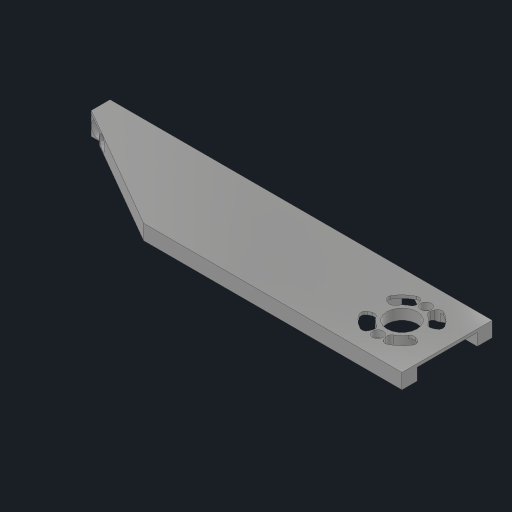
# Autodesk Inventor part: right_hold
Saved by Autodesk Inventor 2023 (Build 270158000, 158)
## iProperties
Created: 2024-05-18
Part Number: right_hold
Material: Nylon 6/6
Document SubType Name: Modeling
Designer: szymo
Density: 1.13 g/cm^3
Appearance: Smooth - Medium Gray
Mass: 11.7755 g
Surface Area: 98.1718 cm^2
Volume: 10.4208 cm^3
Author: szymo
Autodesk Inventor part; units mm, degrees
ref_plane "YZ Plane" through (0, 0, 0) normal (1, 0, 0) x (0, 1, 0)
ref_plane "XZ Plane" through (0, 0, 0) normal (0, 1, 0) x (-1, 0, 0)
ref_plane "XY Plane" through (0, 0, 0) normal (0, 0, 1) x (1, 0, 0)
ref_plane "Work Plane1" through (0, 0, 0) normal (0, 0, 1) x (1, 0, 0)
sketch "Sketch1" plane through (0, 0, 0) normal (0, 0, 1) x (1, 0, 0)
  line L0 (-71, -74) -> (-71, -89) projected
  line L1 (-71, -89) -> (41, -89) projected
  line L2 (41, -89) -> (41, -30.5) projected
  line L3 (41, -30.5) -> (91, -30.5) projected
  line L4 (91, -30.5) -> (91, 30.5) projected
  line L5 (91, 30.5) -> (41, 30.5) projected
  line L6 (41, 30.5) -> (41, 89) projected
  line L7 (41, 89) -> (-71, 89) projected
  line L8 (-71, 89) -> (-71, 74) projected
  line L9 (-71, 74) -> (-87, 74) projected
  line L10 (-87, 74) -> (-87, 89) projected
  line L11 (-87, 89) -> (-91, 89) projected
  line L12 (-91, 89) -> (-91, -89) projected
  line L13 (-91, -89) -> (-87, -89) projected
  line L14 (-87, -89) -> (-87, -74) projected
  line L15 (-87, -74) -> (-71, -74) projected
  line L16 (12, 37) -> (40, 37) projected
  line L17 (41, 37) -> (-86, 37)
  line L18 (-86, 37) -> (-86, 36)
  line L19 (-86, 36) -> (41, 36)
  line L20 (41, 36) -> (41, 37)
  circle A0 centre (-83, 21.5) radius 1.2295 projected
  circle A1 centre (-83, -64.5) radius 1.2295 projected
  circle A2 centre (-83, -21.5) radius 1.2295 projected
  circle A3 centre (-83, 64.5) radius 1.2295 projected
  line L21 (-85, -72) -> (-76, -72) projected
  line L22 (-76, -72) -> (-76, -57) projected
  line L23 (-76, -57) -> (-85, -57) projected
  arc A4 (-87, -55) -> (-85, -57) centre (-85, -55) ccw projected
  line L24 (-87, -55) -> (-87, -31) projected
  arc A5 (-85, -29) -> (-87, -31) centre (-85, -31) ccw projected
  line L25 (-85, -29) -> (-76, -29) projected
  line L26 (-76, -29) -> (-76, -14) projected
  line L27 (-76, -14) -> (-85, -14) projected
  arc A6 (-87, -12) -> (-85, -14) centre (-85, -12) ccw projected
  line L28 (-87, -12) -> (-87, 12) projected
  arc A7 (-85, 14) -> (-87, 12) centre (-85, 12) ccw projected
  line L29 (-85, 14) -> (-76, 14) projected
  line L30 (-76, 14) -> (-76, 29) projected
  line L31 (-76, 29) -> (-85, 29) projected
  arc A8 (-87, 31) -> (-85, 29) centre (-85, 31) ccw projected
  line L32 (-87, 31) -> (-87, 55) projected
  arc A9 (-85, 57) -> (-87, 55) centre (-85, 55) ccw projected
  line L33 (-85, 57) -> (-76, 57) projected
  line L34 (-76, 57) -> (-76, 72) projected
  line L35 (-76, 72) -> (-85, 72) projected
  arc A10 (-87, 74) -> (-85, 72) centre (-85, 74) ccw projected
  line L36 (-87, 74) -> (-87, 89) projected
  line L37 (-91, 89) -> (-87, 89) projected
  line L38 (-91, -89) -> (-91, 89) projected
  line L39 (-91, -89) -> (-87, -89) projected
  line L40 (-87, -89) -> (-87, -74) projected
  arc A11 (-85, -72) -> (-87, -74) centre (-85, -74) ccw projected
  point P0 (0, 0)
  dimension "d1" = 0
  dimension "d2" = 1
  dimension "d11" = 1
  constraints: 8 end point, 2 parallel, 1 horizontal, 1 perpendicular, 1 point on line
  measures "d1" distance between parallel lines of L16 L17
  measures "d2" distance between parallel lines of L16 L19
  measures "d11" distance between parallel lines of L18 L32
ref_plane "Work Plane2" through (11, 8.5, 30) normal (0, 0, 1) x (1, 0, 0)
extrude "Extrusion1" add sketch "Sketch1" along normal up to surface (30 mm away) contours L19 L18 L17 L16 L6
ref_plane "Work Plane3" through (-90.5, 89, 1) normal (0, 1, 0) x (0, 0, 1)
sketch "Sketch3" plane through (-90.5, 89, 1) normal (0, 1, 0) x (0, 0, 1)
  line L0 (3.5, 3.5) -> (-1, 3.5) projected
  line L1 (-1, 3.5) -> (-1, -0.5) projected
  line L2 (-1, -0.5) -> (-4.5, -0.5) projected
  line L3 (-4.5, -0.5) -> (-4.5, -14.5) projected
  line L4 (-4.5, -14.5) -> (4.5, -0.5) projected
  line L5 (4.5, -0.5) -> (3.5, -0.5) projected
  line L6 (3.5, -0.5) -> (3.5, 3.5) projected
  line L7 (29, 4.5) -> (29, 131.5) projected
  line L8 (-1, 131.5) -> (29, 131.5) projected
  line L9 (-1, 131.5) -> (-1, 4.5) projected
  line L10 (-1, 4.5) -> (29, 4.5) projected
  line L11 (3.5, -0.5) -> (30.1547, 45.6673)
  line L12 (30.1547, 45.6673) -> (29, 45.6673)
  line L13 (29, 45.6673) -> (3.5, 1.5)
  point P0 (-1, 90.5)
  point P1 (5.2321, 4.5)
  dimension "d13" = 1
  constraints: 6 end point, 1 midpoint, 1 parallel, 1 perpendicular, 1 point on line
  measures "d13" distance between parallel lines of L13 L11
extrude "Extrusion3" cut sketch "Sketch3" against normal up to next contours L13 L7 L11 L10 | L11 L7 L10
sketch "Sketch7" plane through (41, 36, 0) normal (0, -1, 0) x (1, 0, 0)
  line L0 (-23.0542, 11.42) -> (-22.0416, 11.8701) projected
  arc A0 (-20.7815, 11.4767) -> (-22.0416, 11.8701) centre (-21.6354, 10.9563) ccw projected
  arc A1 (-20.7815, 11.4767) -> (-18.0539, 8.9574) centre (-15, 15) ccw projected
  arc A2 (-17.5618, 7.7324) -> (-18.0539, 8.9574) centre (-18.5049, 8.0649) ccw projected
  line L1 (-17.5618, 7.7324) -> (-17.9302, 6.6874) projected
  arc A3 (-19.3099, 6.1202) -> (-17.9302, 6.6874) centre (-18.8733, 7.0198) ccw projected
  arc A4 (-23.5102, 9.9996) -> (-19.3099, 6.1202) centre (-15, 15) ccw projected
  arc A5 (-23.0542, 11.42) -> (-23.5102, 9.9996) centre (-22.648, 10.5062) ccw projected
  line L2 (-7.9584, 11.8701) -> (-6.9458, 11.42) projected
  arc A6 (-6.4898, 9.9996) -> (-6.9458, 11.42) centre (-7.352, 10.5062) ccw projected
  arc A7 (-10.6901, 6.1202) -> (-6.4898, 9.9996) centre (-15, 15) ccw projected
  arc A8 (-12.0698, 6.6874) -> (-10.6901, 6.1202) centre (-11.1267, 7.0198) ccw projected
  line L3 (-12.0698, 6.6874) -> (-12.4382, 7.7324) projected
  arc A9 (-11.9461, 8.9574) -> (-12.4382, 7.7324) centre (-11.4951, 8.0649) ccw projected
  arc A10 (-11.9461, 8.9574) -> (-9.2185, 11.4767) centre (-15, 15) ccw projected
  arc A11 (-7.9584, 11.8701) -> (-9.2185, 11.4767) centre (-8.3646, 10.9563) ccw projected
  line L4 (-22.0416, 18.1299) -> (-23.0542, 18.58) projected
  arc A12 (-23.5102, 20.0004) -> (-23.0542, 18.58) centre (-22.648, 19.4938) ccw projected
  arc A13 (-19.3099, 23.8798) -> (-23.5102, 20.0004) centre (-15, 15) ccw projected
  arc A14 (-17.9302, 23.3126) -> (-19.3099, 23.8798) centre (-18.8733, 22.9802) ccw projected
  line L5 (-17.9302, 23.3126) -> (-17.5618, 22.2676) projected
  arc A15 (-18.0539, 21.0426) -> (-17.5618, 22.2676) centre (-18.5049, 21.9351) ccw projected
  arc A16 (-18.0539, 21.0426) -> (-20.7815, 18.5233) centre (-15, 15) ccw projected
  arc A17 (-22.0416, 18.1299) -> (-20.7815, 18.5233) centre (-21.6354, 19.0437) ccw projected
  line L6 (-6.9458, 18.58) -> (-7.9584, 18.1299) projected
  arc A18 (-9.2185, 18.5233) -> (-7.9584, 18.1299) centre (-8.3646, 19.0437) ccw projected
  arc A19 (-9.2185, 18.5233) -> (-11.9461, 21.0426) centre (-15, 15) ccw projected
  arc A20 (-12.4382, 22.2676) -> (-11.9461, 21.0426) centre (-11.4951, 21.9351) ccw projected
  line L7 (-12.4382, 22.2676) -> (-12.0698, 23.3126) projected
  arc A21 (-10.6901, 23.8798) -> (-12.0698, 23.3126) centre (-11.1267, 22.9802) ccw projected
  arc A22 (-6.4898, 20.0004) -> (-10.6901, 23.8798) centre (-15, 15) ccw projected
  arc A23 (-6.9458, 18.58) -> (-6.4898, 20.0004) centre (-7.352, 19.4938) ccw projected
  circle A24 centre (-15, 23) radius 1.2295 projected
  circle A25 centre (-15, 7) radius 1.2295 projected
  circle A26 centre (-15, 15) radius 5 projected
  circle A27 centre (-15, 15) radius 14 projected
  circle A28 centre (-15, 15) radius 15 projected
  arc A29 (-23.9413, 20.2537) -> (-23.2572, 18.1231) centre (-22.648, 19.4938) ccw
  line L8 (-23.2572, 18.1231) -> (-22.2447, 17.673)
  arc A30 (-22.2447, 17.673) -> (-20.3545, 18.2631) centre (-21.6354, 19.0437) ccw
  arc A31 (-17.8283, 20.5964) -> (-20.3545, 18.2631) centre (-15, 15) ccw
  arc A32 (-17.8283, 20.5964) -> (-17.0902, 22.4338) centre (-18.5049, 21.9351) ccw
  line L9 (-17.0902, 22.4338) -> (-17.4586, 23.4789)
  arc A33 (-17.4586, 23.4789) -> (-19.5283, 24.3296) centre (-18.8733, 22.9802) ccw
  arc A34 (-19.5283, 24.3296) -> (-23.9413, 20.2537) centre (-15, 15) ccw
  arc A35 (-10.4717, 24.3296) -> (-12.5414, 23.4789) centre (-11.1267, 22.9802) ccw
  line L10 (-12.5414, 23.4789) -> (-12.9098, 22.4338)
  arc A36 (-12.9098, 22.4338) -> (-12.1717, 20.5964) centre (-11.4951, 21.9351) ccw
  arc A37 (-9.6455, 18.2631) -> (-12.1717, 20.5964) centre (-15, 15) ccw
  arc A38 (-9.6455, 18.2631) -> (-7.7553, 17.673) centre (-8.3646, 19.0437) ccw
  line L11 (-7.7553, 17.673) -> (-6.7428, 18.1231)
  arc A39 (-6.7428, 18.1231) -> (-6.0587, 20.2537) centre (-7.352, 19.4938) ccw
  arc A40 (-6.0587, 20.2537) -> (-10.4717, 24.3296) centre (-15, 15) ccw
  arc A41 (-20.3545, 11.7369) -> (-17.8283, 9.4036) centre (-15, 15) ccw
  arc A42 (-20.3545, 11.7369) -> (-22.2447, 12.327) centre (-21.6354, 10.9563) ccw
  line L12 (-22.2447, 12.327) -> (-23.2572, 11.8769)
  arc A43 (-23.2572, 11.8769) -> (-23.9413, 9.7463) centre (-22.648, 10.5062) ccw
  arc A44 (-23.9413, 9.7463) -> (-19.5283, 5.6704) centre (-15, 15) ccw
  arc A45 (-19.5283, 5.6704) -> (-17.4586, 6.5211) centre (-18.8733, 7.0198) ccw
  line L13 (-17.4586, 6.5211) -> (-17.0902, 7.5662)
  arc A46 (-17.0902, 7.5662) -> (-17.8283, 9.4036) centre (-18.5049, 8.0649) ccw
  arc A47 (-12.1717, 9.4036) -> (-9.6455, 11.7369) centre (-15, 15) ccw
  arc A48 (-12.1717, 9.4036) -> (-12.9098, 7.5662) centre (-11.4951, 8.0649) ccw
  line L14 (-12.9098, 7.5662) -> (-12.5414, 6.5211)
  arc A49 (-12.5414, 6.5211) -> (-10.4717, 5.6704) centre (-11.1267, 7.0198) ccw
  arc A50 (-10.4717, 5.6704) -> (-6.0587, 9.7463) centre (-15, 15) ccw
  arc A51 (-6.0587, 9.7463) -> (-6.7428, 11.8769) centre (-7.352, 10.5062) ccw
  line L15 (-6.7428, 11.8769) -> (-7.7553, 12.327)
  arc A52 (-7.7553, 12.327) -> (-9.6455, 11.7369) centre (-8.3646, 10.9563) ccw
  circle A53 centre (-15, 23) radius 1.4
  circle A54 centre (-15, 7) radius 1.4
  point P0 (-41, 0)
  dimension "d21" = 0.5
  dimension "d22" = 0.5
  dimension "d23" = 0.5
  dimension "d24" = 0.5
  dimension "d25" = 2.8
  dimension "d26" = 2.8
  constraints: 48 point on circle, 26 centre point, 16 end point, 2 coincident, 28 other
  measures "d21" radial gap between concentric circles of A13 A34
  measures "d22" radial gap between concentric circles of A22 A40
  measures "d23" radial gap between concentric circles of A1 A41
  measures "d24" radial gap between concentric circles of A10 A47
  measures "d25" diameter of A53
  measures "d26" diameter of A54
extrude "motur" cut sketch "Sketch7" against normal up to next contours L0 A0 A1 A2 L1 A3 A4 A5 | L2 A6 A7 A8 L3 A9 A10 A11 | L4 A12 A13 A14 L5 A15 A16 A17 | L6 A18 A19 A20 L7 A21 A22 A23 | A24 | A25 | A26 | A34 A33 L9 A32 A31 A30 L8 A29 | A40 A39 L11 A38 A37 A36 L10 A35 | A41 A46 L13 A45 A44 A43 L12 A42 | A47 A52 L15 A51 A50 A49 L14 A48 | A53 | A54
sketch "Sketch9" plane through (-86, 36, 0) normal (0, -1, 0) x (1, 0, 0)
  circle A0 centre (112, 23) radius 1.4 projected
  arc A1 (103.0587, 9.7463) -> (107.4717, 5.6704) centre (112, 15) ccw projected
  arc A2 (103.7428, 11.8769) -> (103.0587, 9.7463) centre (104.352, 10.5062) ccw projected
  line L0 (103.7428, 11.8769) -> (104.7553, 12.327) projected
  arc A3 (106.6455, 11.7369) -> (104.7553, 12.327) centre (105.3646, 10.9563) ccw projected
  arc A4 (106.6455, 11.7369) -> (109.1717, 9.4036) centre (112, 15) ccw projected
  arc A5 (109.9098, 7.5662) -> (109.1717, 9.4036) centre (108.4951, 8.0649) ccw projected
  line L1 (109.9098, 7.5662) -> (109.5414, 6.5211) projected
  arc A6 (107.4717, 5.6704) -> (109.5414, 6.5211) centre (108.1267, 7.0198) ccw projected
  arc A7 (120.2572, 18.1231) -> (120.9413, 20.2537) centre (119.648, 19.4938) ccw projected
  line L2 (120.2572, 18.1231) -> (119.2447, 17.673) projected
  arc A8 (117.3545, 18.2631) -> (119.2447, 17.673) centre (118.6354, 19.0437) ccw projected
  arc A9 (117.3545, 18.2631) -> (114.8283, 20.5964) centre (112, 15) ccw projected
  arc A10 (114.0902, 22.4338) -> (114.8283, 20.5964) centre (115.5049, 21.9351) ccw projected
  line L3 (114.0902, 22.4338) -> (114.4586, 23.4789) projected
  arc A11 (116.5283, 24.3296) -> (114.4586, 23.4789) centre (115.8733, 22.9802) ccw projected
  arc A12 (120.9413, 20.2537) -> (116.5283, 24.3296) centre (112, 15) ccw projected
  arc A13 (109.5414, 23.4789) -> (107.4717, 24.3296) centre (108.1267, 22.9802) ccw projected
  line L4 (109.5414, 23.4789) -> (109.9098, 22.4338) projected
  arc A14 (109.1717, 20.5964) -> (109.9098, 22.4338) centre (108.4951, 21.9351) ccw projected
  arc A15 (109.1717, 20.5964) -> (106.6455, 18.2631) centre (112, 15) ccw projected
  arc A16 (104.7553, 17.673) -> (106.6455, 18.2631) centre (105.3646, 19.0437) ccw projected
  line L5 (104.7553, 17.673) -> (103.7428, 18.1231) projected
  arc A17 (103.0587, 20.2537) -> (103.7428, 18.1231) centre (104.352, 19.4938) ccw projected
  arc A18 (107.4717, 24.3296) -> (103.0587, 20.2537) centre (112, 15) ccw projected
  circle A19 centre (112, 7) radius 1.4 projected
  arc A20 (116.5283, 5.6704) -> (120.9413, 9.7463) centre (112, 15) ccw projected
  arc A21 (114.4586, 6.5211) -> (116.5283, 5.6704) centre (115.8733, 7.0198) ccw projected
  line L6 (114.4586, 6.5211) -> (114.0902, 7.5662) projected
  arc A22 (114.8283, 9.4036) -> (114.0902, 7.5662) centre (115.5049, 8.0649) ccw projected
  arc A23 (114.8283, 9.4036) -> (117.3545, 11.7369) centre (112, 15) ccw projected
  arc A24 (119.2447, 12.327) -> (117.3545, 11.7369) centre (118.6354, 10.9563) ccw projected
  line L7 (119.2447, 12.327) -> (120.2572, 11.8769) projected
  arc A25 (120.9413, 9.7463) -> (120.2572, 11.8769) centre (119.648, 10.5062) ccw projected
  circle A26 centre (112, 15) radius 5 projected
  line L8 (41.1673, 30) -> (0, 6.2321) projected
  line L9 (0, 0) -> (0, 6.2321) projected
  line L10 (0, 0) -> (127, 0) projected
  line L11 (127, 0) -> (127, 30) projected
  line L12 (127, 30) -> (41.1673, 30) projected
  line L13 (0, 6.2321) -> (6.5, 6.2321)
  line L14 (6.5, 6.2321) -> (6.5, 0)
  line L15 (6.5, 0) -> (0, 0)
  line L16 (0, 0) -> (0, 6.2321)
  point P0 (86, 0)
  dimension "d31" = 6.5
  constraints: 8 end point, 2 parallel, 1 horizontal, 1 perpendicular, 1 point on line
  measures "d31" distance of L14.end L15.end
extrude "forScrew" add sketch "Sketch9" along normal blind 6.5 contours L13 L14 L10 L9
sketch "Sketch10" plane through (41, 36, 0) normal (0, -1, 0) x (1, 0, 0)
  line L0 (-120.5, 6.2321) -> (-120.5, 0) projected
  line L1 (-120.5, 0) -> (0, 0) projected
  line L2 (0, 0) -> (0, 30) projected
  line L3 (0, 30) -> (-85.8327, 30) projected
  line L4 (-85.8327, 30) -> (-127, 6.2321) projected
  line L5 (-127, 6.2321) -> (-120.5, 6.2321) projected
  circle A0 centre (-15, 23) radius 1.4 projected
  arc A1 (-23.9413, 9.7463) -> (-19.5283, 5.6704) centre (-15, 15) ccw projected
  arc A2 (-23.2572, 11.8769) -> (-23.9413, 9.7463) centre (-22.648, 10.5062) ccw projected
  line L6 (-23.2572, 11.8769) -> (-22.2447, 12.327) projected
  arc A3 (-20.3545, 11.7369) -> (-22.2447, 12.327) centre (-21.6354, 10.9563) ccw projected
  arc A4 (-20.3545, 11.7369) -> (-17.8283, 9.4036) centre (-15, 15) ccw projected
  arc A5 (-17.0902, 7.5662) -> (-17.8283, 9.4036) centre (-18.5049, 8.0649) ccw projected
  line L7 (-17.0902, 7.5662) -> (-17.4586, 6.5211) projected
  arc A6 (-19.5283, 5.6704) -> (-17.4586, 6.5211) centre (-18.8733, 7.0198) ccw projected
  arc A7 (-6.7428, 18.1231) -> (-6.0587, 20.2537) centre (-7.352, 19.4938) ccw projected
  line L8 (-6.7428, 18.1231) -> (-7.7553, 17.673) projected
  arc A8 (-9.6455, 18.2631) -> (-7.7553, 17.673) centre (-8.3646, 19.0437) ccw projected
  arc A9 (-9.6455, 18.2631) -> (-12.1717, 20.5964) centre (-15, 15) ccw projected
  arc A10 (-12.9098, 22.4338) -> (-12.1717, 20.5964) centre (-11.4951, 21.9351) ccw projected
  line L9 (-12.9098, 22.4338) -> (-12.5414, 23.4789) projected
  arc A11 (-10.4717, 24.3296) -> (-12.5414, 23.4789) centre (-11.1267, 22.9802) ccw projected
  arc A12 (-6.0587, 20.2537) -> (-10.4717, 24.3296) centre (-15, 15) ccw projected
  arc A13 (-17.4586, 23.4789) -> (-19.5283, 24.3296) centre (-18.8733, 22.9802) ccw projected
  line L10 (-17.4586, 23.4789) -> (-17.0902, 22.4338) projected
  arc A14 (-17.8283, 20.5964) -> (-17.0902, 22.4338) centre (-18.5049, 21.9351) ccw projected
  arc A15 (-17.8283, 20.5964) -> (-20.3545, 18.2631) centre (-15, 15) ccw projected
  arc A16 (-22.2447, 17.673) -> (-20.3545, 18.2631) centre (-21.6354, 19.0437) ccw projected
  line L11 (-22.2447, 17.673) -> (-23.2572, 18.1231) projected
  arc A17 (-23.9413, 20.2537) -> (-23.2572, 18.1231) centre (-22.648, 19.4938) ccw projected
  arc A18 (-19.5283, 24.3296) -> (-23.9413, 20.2537) centre (-15, 15) ccw projected
  circle A19 centre (-15, 7) radius 1.4 projected
  arc A20 (-10.4717, 5.6704) -> (-6.0587, 9.7463) centre (-15, 15) ccw projected
  arc A21 (-12.5414, 6.5211) -> (-10.4717, 5.6704) centre (-11.1267, 7.0198) ccw projected
  line L12 (-12.5414, 6.5211) -> (-12.9098, 7.5662) projected
  arc A22 (-12.1717, 9.4036) -> (-12.9098, 7.5662) centre (-11.4951, 8.0649) ccw projected
  arc A23 (-12.1717, 9.4036) -> (-9.6455, 11.7369) centre (-15, 15) ccw projected
  arc A24 (-7.7553, 12.327) -> (-9.6455, 11.7369) centre (-8.3646, 10.9563) ccw projected
  line L13 (-7.7553, 12.327) -> (-6.7428, 11.8769) projected
  arc A25 (-6.0587, 9.7463) -> (-6.7428, 11.8769) centre (-7.352, 10.5062) ccw projected
  circle A26 centre (-15, 15) radius 5 projected
  line L14 (-120.5, 6.2321) -> (-120.5, 9.9848)
  line L15 (-120.5, 9.9848) -> (-116.1699, 12.4848)
  line L16 (-116.1699, 12.4848) -> (-113.6699, 8.1547)
  line L17 (-113.6699, 8.1547) -> (-118, 5.6547)
  line L18 (-118, 5.6547) -> (-120.5, 9.9848)
  line L19 (-113.6699, 8.1547) -> (-113.6699, 0)
  line L20 (-113.6699, 8.1547) -> (-113.6699, 13.9282)
  point P0 (-41, 0)
  dimension "d34" = 5
  dimension "d35" = 5
  constraints: 14 end point, 4 point on line, 2 parallel, 2 perpendicular, 2 vertical
  measures "d34" distance of L14.end L15.end
  measures "d35" distance of L15.end L16.end
extrude "for insert" add sketch "Sketch10" along normal blind 4 contours L14 L18 L17 L19 L1 L0 | L4 L16 L17 L18 | L4 L20 L16
sketch "Sketch15" plane through (41, 36, 0) normal (0, -1, 0) x (1, 0, 0)
  line L0 (-85.8327, 30) -> (-113.6699, 13.9282) projected
  line L1 (0, 30) -> (-85.8327, 30) projected
  line L2 (0, 0) -> (0, 30) projected
  line L3 (-113.6699, 0) -> (0, 0) projected
  line L4 (-113.6699, 0) -> (-113.6699, 13.9282) projected
  line L5 (-113.6699, 7) -> (-73.8327, 30)
  line L6 (-85.8327, 30) -> (0, 30) projected
  circle A0 centre (-15, 15) radius 15 projected
  circle A1 centre (-15, 15) radius 15 projected
  circle A2 centre (-15, 15) radius 15 projected
  line L7 (-23.0542, 11.42) -> (-22.0416, 11.8701) projected
  arc A3 (-20.7815, 11.4767) -> (-22.0416, 11.8701) centre (-21.6354, 10.9563) ccw projected
  arc A4 (-20.7815, 11.4767) -> (-18.0539, 8.9574) centre (-15, 15) ccw projected
  arc A5 (-17.5618, 7.7324) -> (-18.0539, 8.9574) centre (-18.5049, 8.0649) ccw projected
  line L8 (-17.5618, 7.7324) -> (-17.9302, 6.6874) projected
  arc A6 (-19.3099, 6.1202) -> (-17.9302, 6.6874) centre (-18.8733, 7.0198) ccw projected
  arc A7 (-23.5102, 9.9996) -> (-19.3099, 6.1202) centre (-15, 15) ccw projected
  arc A8 (-23.0542, 11.42) -> (-23.5102, 9.9996) centre (-22.648, 10.5062) ccw projected
  line L9 (-7.9584, 11.8701) -> (-6.9458, 11.42) projected
  arc A9 (-6.4898, 9.9996) -> (-6.9458, 11.42) centre (-7.352, 10.5062) ccw projected
  arc A10 (-10.6901, 6.1202) -> (-6.4898, 9.9996) centre (-15, 15) ccw projected
  arc A11 (-12.0698, 6.6874) -> (-10.6901, 6.1202) centre (-11.1267, 7.0198) ccw projected
  line L10 (-12.0698, 6.6874) -> (-12.4382, 7.7324) projected
  arc A12 (-11.9461, 8.9574) -> (-12.4382, 7.7324) centre (-11.4951, 8.0649) ccw projected
  arc A13 (-11.9461, 8.9574) -> (-9.2185, 11.4767) centre (-15, 15) ccw projected
  arc A14 (-7.9584, 11.8701) -> (-9.2185, 11.4767) centre (-8.3646, 10.9563) ccw projected
  line L11 (-22.0416, 18.1299) -> (-23.0542, 18.58) projected
  arc A15 (-23.5102, 20.0004) -> (-23.0542, 18.58) centre (-22.648, 19.4938) ccw projected
  arc A16 (-19.3099, 23.8798) -> (-23.5102, 20.0004) centre (-15, 15) ccw projected
  arc A17 (-17.9302, 23.3126) -> (-19.3099, 23.8798) centre (-18.8733, 22.9802) ccw projected
  line L12 (-17.9302, 23.3126) -> (-17.5618, 22.2676) projected
  arc A18 (-18.0539, 21.0426) -> (-17.5618, 22.2676) centre (-18.5049, 21.9351) ccw projected
  arc A19 (-18.0539, 21.0426) -> (-20.7815, 18.5233) centre (-15, 15) ccw projected
  arc A20 (-22.0416, 18.1299) -> (-20.7815, 18.5233) centre (-21.6354, 19.0437) ccw projected
  line L13 (-6.9458, 18.58) -> (-7.9584, 18.1299) projected
  arc A21 (-9.2185, 18.5233) -> (-7.9584, 18.1299) centre (-8.3646, 19.0437) ccw projected
  arc A22 (-9.2185, 18.5233) -> (-11.9461, 21.0426) centre (-15, 15) ccw projected
  arc A23 (-12.4382, 22.2676) -> (-11.9461, 21.0426) centre (-11.4951, 21.9351) ccw projected
  line L14 (-12.4382, 22.2676) -> (-12.0698, 23.3126) projected
  arc A24 (-10.6901, 23.8798) -> (-12.0698, 23.3126) centre (-11.1267, 22.9802) ccw projected
  arc A25 (-6.4898, 20.0004) -> (-10.6901, 23.8798) centre (-15, 15) ccw projected
  arc A26 (-6.9458, 18.58) -> (-6.4898, 20.0004) centre (-7.352, 19.4938) ccw projected
  circle A27 centre (-15, 23) radius 1.2295 projected
  circle A28 centre (-15, 7) radius 1.2295 projected
  circle A29 centre (-15, 15) radius 5 projected
  circle A30 centre (-15, 15) radius 14 projected
  line L15 (0, 30) -> (-5, 30)
  line L16 (-5, 30) -> (-5, 25)
  line L17 (-5, 25) -> (0, 25)
  line L18 (0, 25) -> (0, 30)
  line L19 (0, 0) -> (-127, 0) projected
  line L20 (0, 0) -> (-5, 0)
  line L21 (-5, 0) -> (-5, 5)
  line L22 (-5, 5) -> (0, 5)
  line L23 (0, 5) -> (0, 0)
  line L24 (-30, 30) -> (-30, 0)
  line L25 (-113.6699, 6) -> (-30, 6)
  line L26 (-127, 6.2321) -> (-85.8327, 30) projected
  line L27 (-96.225, 24) -> (-30, 24)
  line L28 (-86.9898, 22.4037) -> (-67.4406, 6)
  line L29 (-79.5578, 24) -> (-58.1063, 6)
  line L30 (-62.7734, 6) -> (-84.225, 24) construction
  line L31 (-22.8495, 0) -> (-58.6021, 30)
  line L32 (-34.6672, 6) -> (-56.1187, 24) construction
  line L33 (-60.7859, 24) -> (-39.3343, 6)
  line L34 (-100.3298, 14.7019) -> (-89.9594, 6) construction
  line L35 (-94.6265, 6) -> (-103.0947, 13.1056)
  line L36 (-97.565, 16.2981) -> (-85.2922, 6)
  line L37 (-56.2186, 28) -> (-5, 28)
  line L38 (-25.233, 2) -> (-5, 2)
  line L39 (-5, 28) -> (-5, 30)
  line L40 (-5, 30) -> (-58.6021, 30)
  line L41 (-5, 28) -> (-56.2186, 28)
  line L42 (-30, 30) -> (-25, 30)
  line L43 (-25, 30) -> (-25, 25)
  line L44 (-25, 25) -> (-30, 25)
  line L45 (-30, 25) -> (-30, 30)
  point P0 (-41, 0)
  point P1 (-3.8197, 25)
  point P2 (-30, 28)
  point P3 (-5, 26.1803)
  point P4 (-3.8197, 5)
  point P5 (-5, 3.8197)
  point P6 (-30, 28)
  point P7 (-25, 28)
  dimension "d40" = 6
  dimension "d45" = 5
  dimension "d46" = 5
  dimension "d47" = 5
  dimension "d48" = 5
  dimension "d50" = 6
  dimension "d53" = 6
  dimension "d57" = 3
  dimension "d58" = 3
  dimension "d59" = 40
  dimension "d60" = 3
  dimension "d61" = 3
  dimension "d62" = 13.34
  dimension "d63" = 13.34
  dimension "d64" = 3
  dimension "d65" = 3
  dimension "d66" = 2
  dimension "d67" = 2
  dimension "d70" = 5
  dimension "d71" = 5
  constraints: 58 end point, 24 point on line, 18 parallel, 6 perpendicular, 4 horizontal, 1 collinear, 1 tangent, 11 other
  measures "d40" distance between parallel lines of L0 L5
  measures "d45" distance of L17.end L16.end
  measures "d46" distance of L16.end L15.end
  measures "d47" distance of L21.end L22.end
  measures "d48" distance of L20.end L21.end
  measures "d53" distance between parallel lines of L1 L27
  measures "d57" distance between parallel lines of L30 L29
  measures "d58" distance between parallel lines of L30 L28
  measures "d59" angle of L27 L30
  measures "d60" distance between parallel lines of L32 L31
  measures "d61" distance between parallel lines of L32 L33
  measures "d62" horizontal distance of L34.start L5.start
  measures "d63" horizontal distance of L28.start L34.start
  measures "d64" distance between parallel lines of L34 L36
  measures "d65" distance between parallel lines of L34 L35
  measures "d66" distance between parallel lines of L1 L37
  measures "d67" distance between parallel lines of L38 L19
  measures "d70" distance of L43.end L44.end
  measures "d71" distance of L42.end L43.end
extrude "zeberka" add sketch "Sketch15" along normal blind 4 contours L1 L5 L27 L0 | L27 L5 L4 L0 | L1 L31 L27 L5 | L27 L29 L25 L28 L5 | L1 L24 L37 L31 | L1 L43 L37 L24 | L25 L24 L3 L4 | L5 L36 L25 L35 | L27 L31 L25 L33 | L1 A0 L37 L43 | L37 L43 A0 L44 L24 | L1 L16 L37 A0 | A0 L37 A30 | L31 L3 L24 | L1 L2 L17 A0 L16 | L43 L44 A0 | L38 A0 L3 L31 | A0 L17 L16 | L37 A30 | L38 A30 A0 | A0 L38 L21 L3 | L38 A30 | L21 A0 L22 L2 L3 | L21 L22 A0
sketch "Sketch17" plane through (-15.2186, 36, 28) normal (0, -1, 0) x (1, 0, 0)
  line L0 (51.2186, -23) -> (56.2186, -23) projected
  line L1 (56.2186, -23) -> (56.2186, -3) projected
  line L2 (56.2186, -3) -> (51.2186, -3) projected
  line L3 (51.2186, -3) -> (51.2186, 0) projected
  line L4 (51.2186, 0) -> (31.2186, 0) projected
  line L5 (31.2186, 0) -> (31.2186, -3) projected
  line L6 (31.2186, -3) -> (26.2186, -3) projected
  line L7 (26.2186, -3) -> (26.2186, 0) projected
  line L8 (26.2186, 0) -> (0, 0) projected
  line L9 (0, 0) -> (30.9856, -26) projected
  line L10 (30.9856, -26) -> (51.2186, -26) projected
  line L11 (51.2186, -26) -> (51.2186, -23) projected
  circle A0 centre (41.2186, -13) radius 5 projected
  arc A1 (45.7468, -22.3296) -> (50.1598, -18.2537) centre (41.2186, -13) ccw projected
  arc A2 (43.6772, -21.4789) -> (45.7468, -22.3296) centre (45.0919, -20.9802) ccw projected
  line L12 (43.6772, -21.4789) -> (43.3088, -20.4338) projected
  arc A3 (44.0469, -18.5964) -> (43.3088, -20.4338) centre (44.7235, -19.9351) ccw projected
  arc A4 (44.0469, -18.5964) -> (46.5731, -16.2631) centre (41.2186, -13) ccw projected
  arc A5 (48.4633, -15.673) -> (46.5731, -16.2631) centre (47.854, -17.0437) ccw projected
  line L13 (48.4633, -15.673) -> (49.4758, -16.1231) projected
  arc A6 (50.1598, -18.2537) -> (49.4758, -16.1231) centre (48.8666, -17.4938) ccw projected
  circle A7 centre (41.2186, -21) radius 1.4 projected
  arc A8 (38.76, -4.5211) -> (36.6903, -3.6704) centre (37.3453, -5.0198) ccw projected
  line L14 (38.76, -4.5211) -> (39.1283, -5.5662) projected
  arc A9 (38.3902, -7.4036) -> (39.1283, -5.5662) centre (37.7137, -6.0649) ccw projected
  arc A10 (38.3902, -7.4036) -> (35.864, -9.7369) centre (41.2186, -13) ccw projected
  arc A11 (33.9739, -10.327) -> (35.864, -9.7369) centre (34.5831, -8.9563) ccw projected
  line L15 (33.9739, -10.327) -> (32.9613, -9.8769) projected
  arc A12 (32.2773, -7.7463) -> (32.9613, -9.8769) centre (33.5706, -8.5062) ccw projected
  arc A13 (36.6903, -3.6704) -> (32.2773, -7.7463) centre (41.2186, -13) ccw projected
  arc A14 (49.4758, -9.8769) -> (50.1598, -7.7463) centre (48.8666, -8.5062) ccw projected
  line L16 (49.4758, -9.8769) -> (48.4633, -10.327) projected
  arc A15 (46.5731, -9.7369) -> (48.4633, -10.327) centre (47.854, -8.9563) ccw projected
  arc A16 (46.5731, -9.7369) -> (44.0469, -7.4036) centre (41.2186, -13) ccw projected
  arc A17 (43.3088, -5.5662) -> (44.0469, -7.4036) centre (44.7235, -6.0649) ccw projected
  line L17 (43.3088, -5.5662) -> (43.6772, -4.5211) projected
  arc A18 (45.7468, -3.6704) -> (43.6772, -4.5211) centre (45.0919, -5.0198) ccw projected
  arc A19 (50.1598, -7.7463) -> (45.7468, -3.6704) centre (41.2186, -13) ccw projected
  arc A20 (32.2773, -18.2537) -> (36.6903, -22.3296) centre (41.2186, -13) ccw projected
  arc A21 (32.9613, -16.1231) -> (32.2773, -18.2537) centre (33.5706, -17.4938) ccw projected
  line L18 (32.9613, -16.1231) -> (33.9739, -15.673) projected
  arc A22 (35.864, -16.2631) -> (33.9739, -15.673) centre (34.5831, -17.0437) ccw projected
  arc A23 (35.864, -16.2631) -> (38.3902, -18.5964) centre (41.2186, -13) ccw projected
  arc A24 (39.1283, -20.4338) -> (38.3902, -18.5964) centre (37.7137, -19.9351) ccw projected
  line L19 (39.1283, -20.4338) -> (38.76, -21.4789) projected
  arc A25 (36.6903, -22.3296) -> (38.76, -21.4789) centre (37.3453, -20.9802) ccw projected
  circle A26 centre (41.2186, -5) radius 1.4 projected
  line L20 (39.1283, -5.5662) -> (38.76, -4.5211) projected
  line L21 (38.9288, -5) -> (43.592, -5) construction
  arc A27 (38.76, -4.5211) -> (36.6903, -3.6704) centre (37.3453, -5.0198) ccw projected
  circle A28 centre (41.2186, -5) radius 1.4 projected
  line L22 (37.8292, -3.6) -> (44.608, -3.6) construction
  line L23 (37.8292, -3.6) -> (31.2186, 0)
  line L24 (51.2186, 0) -> (51.2186, -3) projected
  line L25 (44.608, -3.6) -> (51.2186, 0)
  line L26 (39.1757, -6.4) -> (43.2614, -6.4) construction
  circle A29 centre (41.2186, -13) radius 6.2705
  line L27 (34.9481, -13) -> (47.4891, -13) construction
  line L28 (38.9288, -21) -> (43.592, -21) construction
  line L29 (37.8292, -22.4) -> (44.608, -22.4) construction
  line L30 (37.8292, -22.4) -> (31.2186, -26)
  line L31 (44.608, -22.4) -> (51.2186, -26)
  line L32 (39.1757, -19.6) -> (43.2614, -19.6) construction
  point P0 (15.2186, -28)
  point P1 (37.8292, -3.6)
  point P2 (35.864, -9.7369)
  point P3 (35.864, -16.2631)
  point P4 (46.5731, -16.2631)
  point P5 (46.5731, -9.7369)
  constraints: 22 end point, 7 point on circle, 7 symmetric about line, 4 horizontal, 2 point on line, 2 tangent, 1 centre point, 1 coincident, 1 concentric, 1 midpoint
extrude "for motor hold" add sketch "Sketch17" along normal blind 2.5 contours L10 L30 A25 L19 A24 A29 A3 L12 A2 L31 | L25 A18 L17 A17 A29 A9 L14 A8 L23 L4 | A29 A23 A10 A16 A4
sketch "Sketch18" plane through (-15.2186, 33.5, 28) normal (0, -1, 0) x (1, 0, 0)
  line L0 (31.2186, 0) -> (37.8292, -3.6) projected
  arc A0 (38.76, -4.5211) -> (37.8292, -3.6) centre (37.3453, -5.0198) ccw projected
  line L1 (38.76, -4.5211) -> (39.1283, -5.5662) projected
  arc A1 (38.3902, -7.4036) -> (39.1283, -5.5662) centre (37.7137, -6.0649) ccw projected
  arc A2 (38.3902, -7.4036) -> (38.3902, -18.5964) centre (41.2186, -13) ccw projected
  arc A3 (39.1283, -20.4338) -> (38.3902, -18.5964) centre (37.7137, -19.9351) ccw projected
  line L2 (39.1283, -20.4338) -> (38.76, -21.4789) projected
  arc A4 (37.8292, -22.4) -> (38.76, -21.4789) centre (37.3453, -20.9802) ccw projected
  line L3 (37.8292, -22.4) -> (31.2186, -26) projected
  line L4 (51.2186, -26) -> (31.2186, -26) projected
  line L5 (51.2186, -26) -> (44.608, -22.4) projected
  arc A5 (43.6772, -21.4789) -> (44.608, -22.4) centre (45.0919, -20.9802) ccw projected
  line L6 (43.6772, -21.4789) -> (43.3088, -20.4338) projected
  arc A6 (44.0469, -18.5964) -> (43.3088, -20.4338) centre (44.7235, -19.9351) ccw projected
  arc A7 (44.0469, -18.5964) -> (44.0469, -7.4036) centre (41.2186, -13) ccw projected
  arc A8 (43.3088, -5.5662) -> (44.0469, -7.4036) centre (44.7235, -6.0649) ccw projected
  line L7 (43.3088, -5.5662) -> (43.6772, -4.5211) projected
  arc A9 (44.608, -3.6) -> (43.6772, -4.5211) centre (45.0919, -5.0198) ccw projected
  line L8 (44.608, -3.6) -> (51.2186, 0) projected
  line L9 (31.2186, 0) -> (51.2186, 0) projected
  circle A10 centre (41.2186, -13) radius 5 projected
  circle A11 centre (41.2186, -21) radius 1.4 projected
  circle A12 centre (41.2186, -5) radius 1.4 projected
  circle A13 centre (41.2186, -5) radius 1.4 projected
  circle A14 centre (41.2186, -21) radius 1.4 projected
  point P0 (15.2186, -28)
  constraints: 2 coincident
hole "Hole1" at (26, 33.5, 23) at (26, 33.5, 7) direction (0, 1, 0) diameter 3.6 end through all countersink diameter 6 countersink angle 90 clearance for "Countersunk Flat Head Screw ISO 2009/7046" size "M3" standard "ISO"
sketch "Sketch19" plane through (41, 32, 0) normal (0, -1, 0) x (1, 0, 0)
  line L0 (0, 25) -> (0, 30) projected
  line L1 (0, 30) -> (-85.8327, 30) projected
  line L2 (-85.8327, 30) -> (-120.5, 9.9848) projected
  line L3 (-113.6699, 6) -> (-113.6699, 7) projected
  line L4 (-113.6699, 7) -> (-103.0947, 13.1056) projected
  line L5 (-103.0947, 13.1056) -> (-94.6265, 6) projected
  line L6 (-94.6265, 6) -> (-113.6699, 6) projected
  line L7 (0, 0) -> (0, 5) projected
  line L8 (0, 5) -> (-5, 5) projected
  line L9 (-5, 5) -> (-5, 2) projected
  line L10 (-5, 2) -> (-25.233, 2) projected
  line L11 (-25.233, 2) -> (-56.2186, 28) projected
  line L12 (-56.2186, 28) -> (-30, 28) projected
  line L13 (-30, 28) -> (-30, 25) projected
  line L14 (-30, 25) -> (-25, 25) projected
  line L15 (-25, 25) -> (-25, 28) projected
  line L16 (-25, 28) -> (-5, 28) projected
  line L17 (-5, 28) -> (-5, 25) projected
  line L18 (-5, 25) -> (0, 25) projected
  line L19 (-58.1063, 6) -> (-79.5578, 24) projected
  line L20 (-79.5578, 24) -> (-60.7859, 24) projected
  line L21 (-60.7859, 24) -> (-39.3343, 6) projected
  line L22 (-39.3343, 6) -> (-58.1063, 6) projected
  line L23 (-67.4406, 6) -> (-85.2922, 6) projected
  line L24 (-85.2922, 6) -> (-97.565, 16.2981) projected
  line L25 (-97.565, 16.2981) -> (-86.9898, 22.4037) projected
  line L26 (-86.9898, 22.4037) -> (-67.4406, 6) projected
  line L27 (-32.8343, 0) -> (-39.3343, 0)
  line L28 (-39.3343, 0) -> (-39.3343, 6)
  line L29 (-39.3343, 6) -> (-32.8343, 6)
  line L30 (-32.8343, 6) -> (-32.8343, 0)
  line L31 (-32.8343, 6) -> (-30, 6)
  line L32 (-56.2186, 28) -> (-25.233, 2) projected
  line L33 (-30, 6) -> (-22.8495, 0)
  line L34 (-120.5, 0) -> (0, 0) projected
  line L35 (-120.5, 9.9848) -> (-120.5, 6.2321) projected
  line L36 (-120.5, 0) -> (-120.5, 6.2321) projected
  line L37 (-30, 6) -> (-30, -0.1684)
  point P0 (-41, 0)
  point P1 (-30, 0)
  dimension "d82" = 6.5
  constraints: 14 end point, 2 horizontal, 2 parallel, 2 perpendicular, 2 point on line
  measures "d82" distance of L21.end L29.end
extrude "Extrusion12" add sketch "Sketch19" along normal blind 6.5 contours L28 L29 L30 L27 | L30 L31 L37 L34
sketch "Sketch20" plane through (1.6657, 32, 6) normal (0, 0, 1) x (1, 0, 0)
  line L0 (9.3343, 0) -> (9.3343, -6.5)
  line L1 (9.3343, 0) -> (0, -6.5)
  point P0 (-1.6657, -32)
  point P1 (4.6672, -3.25)
  constraints: 4 end point, 1 midpoint
hole "Hole2" at (6.3328, 28.75, 6) direction (0, 0, -1) diameter 3.6 end through all countersink diameter 6.5 countersink angle 90 clearance for "Countersunk Flat Head Screw ISO 2009/7046" size "M3" standard "ISO"
sketch "Sketch21" plane through (-86, 29.5, 6.2321) normal (0, 0, 1) x (1, 0, 0)
  line L0 (0, 6.5) -> (6.5, 6.5) projected
  line L1 (0, 6.5) -> (0, 0) projected
  line L2 (6.5, 0) -> (0, 0) projected
  line L3 (6.5, 2.5) -> (6.5, 0) projected
  line L4 (6.5, 6.5) -> (6.5, 2.5) projected
  line L5 (0, 6.5) -> (6.5, 0)
  line L6 (0, 0) -> (6.5, 0) projected
  line L7 (6.5, 6.5) -> (0, 0)
  point P0 (86, -29.5)
  point P1 (3.25, 3.25)
  constraints: 4 end point, 1 midpoint, 1 perpendicular
hole "Hole3" at (-82.75, 32.75, 6.2321) direction (0, 0, -1) diameter 3.6 end through all countersink diameter 6.5 countersink angle 90 clearance for "Countersunk Flat Head Screw ISO 2009/7046" size "M3" standard "ISO"
sketch "Sketch22" plane through (-79.5, 32, 9.9848) normal (-0.5, 0, 0.8660254) x (0.8660254, 0, 0.5)
  line L0 (-7.5056, 5) -> (40.0303, 5) projected
  line L1 (-7.5056, 4) -> (-7.5056, 5) projected
  line L2 (0, 4) -> (-7.5056, 4) projected
  line L3 (0, 4) -> (0, 0) projected
  line L4 (40.0303, 0) -> (0, 0) projected
  line L5 (40.0303, 5) -> (40.0303, 0) projected
  line L6 (0, 0) -> (5, 0)
  line L7 (5, 0) -> (5, 5)
  line L8 (5, 5) -> (0, 5)
  line L9 (0, 5) -> (0, 0)
  line L10 (0, 0) -> (5, 5)
  line L11 (5, 0) -> (0, 5)
  point P0 (63.8566, -32)
  point P1 (2.5, 2.5)
  dimension "d99" = 5
  dimension "d100" = 5
  constraints: 12 end point, 2 parallel, 1 horizontal, 1 midpoint, 1 perpendicular
  measures "d99" distance of L8.end L7.end
  measures "d100" distance of L7.end L6.end
hole "Hole4" at (-77.3349, 34.5, 11.2348) direction (0.5, 0, -0.8660254) diameter 4 depth 5.5 counterbore diameter 4.6 counterbore depth 1.5
equation "\"d50\" = d40"
equation "\"d53\" = d40"
equation "\"d57\" = 0.5 * d40"
equation "\"d58\" = d57"
equation "\"d60\" = 0.5 * d40"
equation "\"d61\" = d60"
equation "\"d62\" = d63"
equation "\"d64\" = 0.5 * d40"
equation "\"d65\" = d64"
equation "\"d67\" = d66"
body "Solid1"
